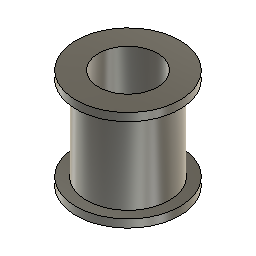
1 x 1 Cable Duct (Autodesk Fusion 360 design; units mm, degrees)
Autodesk Fusion 360 part; units mm, degrees
sketch "Walls" plane through (0, 0, 0) normal (0, 1, 0) x (1, 0, 0)
  line L0 (0, 0) -> (0, -25.4) construction
  line L1 (10.646, 2.4) -> (10.646, -25.4)
  line L2 (10.646, -25.4) -> (12.446, -25.4)
  line L3 (12.446, -25.4) -> (12.446, 0)
  line L4 (12.446, 0) -> (15.621, 0)
  line L5 (15.621, 0) -> (15.621, 2.4)
  line L6 (15.621, 2.4) -> (10.646, 2.4)
  line L7 (10.646, 2.4) -> (8.846, 2.4)
  line L8 (8.846, 2.4) -> (8.846, -27.8)
  line L9 (8.846, -27.8) -> (15.621, -27.8)
  line L10 (15.621, -27.8) -> (15.621, -25.4)
  line L11 (15.621, -25.4) -> (10.646, -25.4)
  line L12 (10.646, 1.2) -> (11.846, 0)
  line L13 (11.846, 0) -> (10.646, -1.2)
  dimension "d56" = 25.4
  dimension "d57" = 2.4
  dimension "d58" = 1.8
  dimension "d59" = 12.446
  dimension "d60" = 3.175
  dimension "d61" = 1.2
  dimension "d62" = 1.2
  constraint parallel L0 L1
  constraint perpendicular L0 L2
  constraint perpendicular L2 L3
  constraint perpendicular L0 L4
  constraint perpendicular L4 L5
  constraint horizontal L6
  constraint coincident L0.start origin
  constraint coincident L0.end L2
  constraint perpendicular L1 L7
  constraint perpendicular L6 L8
  constraint perpendicular L1 L9
  constraint perpendicular L9 L10
  constraint collinear L5 L10
  constraint equal L5 L10
  constraint horizontal L11
  constraint coincident L1 L12.start
  constraint coincident L1 L13.end
  constraint equal L12 L13
  constraint perpendicular L12 L13
  constraint coincident L0.start L4
  measures "d56" distance of L0.start L0.end
  measures "d57" distance of L4.end L5.end
  measures "d58" distance of L1.end L2.end
  measures "d59" distance of L0 L3
  measures "d60" distance of L3.end L4.end
  measures "d61" distance of L1.start L12.start
  measures "d62" distance of L1 L12.end
revolve "Revolve1" add sketch "Walls" angle 360 about axis through (0, 0, 0) along (0, 0, 1) contours L1 L2 L3 L4 L5 L6 L11 L12 L13 makes body 1 in component "Outer"
revolve "Revolve1'" add sketch "Walls" angle 360 about axis through (0, 0, 0) along (0, 0, 1) separate body contours L1 L2 L7 L8 L9 L10 L11 | L1 L12 L13 makes body 2 in component "Inner"
move_face "OffsetFaces1" offset -0.127 5 faces at (10.6328, -0.5307, 9.2667) (11.4318, -0.5705, 0.4) (11.3891, -1.1397, -0.4) (10.5931, -1.06, -1.6) (9.9734, -0.9684, -2.4) on bodies 2 in component "Inner"
sketch "Cutouts" plane through (0, 0, -2.273) normal (0, 0, -1) x (1, 0, 0)
  circle A0 centre (0, 0) radius 8.846
  circle A1 centre (0, 0) radius 10.519
  circle A2 centre (0, 0) radius 8.846 construction
  circle A3 centre (0, 0) radius 15.621 construction
  line L0 (-1.2, 15.621) -> (1.2, 15.621)
  line L1 (1.2, 15.621) -> (1.2, 8.7642)
  line L2 (1.2, 8.7642) -> (-1.2, 8.7642)
  line L3 (-1.2, 8.7642) -> (-1.2, 15.621)
  line L4 (0, 0) -> (0, 8.846) construction
  dimension "d66" = 2.4
  constraint horizontal L0
  constraint vertical L1
  constraint horizontal L2
  constraint vertical L3
  constraint coincident A0.centre A1.centre
  constraint coincident A2 L4.end
  constraint perpendicular L2 L4
  constraint tangent A3 L0
  constraint coincident A2 L2.end
  measures "d66" distance of L0.start L0.end
extrude "Extrude1" cut sketch "Cutouts" against normal blind 12.7 contours A0 L2 | A0 A1 L1 L3 | A1 L0 L1 L3 picked at (0.1337, 8.7885) picked at (-0.9337, 9.3505) bodies 2 in component "Inner"
pattern_circular "C-Pattern1" count 6 over 360 about axis through (0, 0, 0) along (0, 0, 1) of "Extrude1" in component "Inner"
component "Outer" placed x (1, 0, 0) y (0, 1, 0) z (0, 0, 1) at (0, 0, 0)
component "Inner" placed x (1, 0, 0) y (0, 1, 0) z (0, 0, 1) at (0, 0, 0)
equation "DIAMETER = 1 in - 0.02 in" comment "Diameter of ducting"
equation "LENGTH = 1 in" comment "Thickness flange to flange"
equation "PRINTER_TOLERANCE = 0.005 in" comment "Tolerance for printer"
equation "FLANGE = 0.125 in"
equation "SLOT_WIDTH = 2.4 mm" comment "Width of slots for flange flexibility"
equation "SLOT_DEPTH = LENGTH * 0.5" comment "Depth of slot from flange"
equation "FLANGE_THICKNESS = 2.4 mm" comment "Thickness of flange top and bottom"
equation "FLANGE_OVERHANGE = 45 deg" comment "Angle of the compliant flange side"
equation "WALL = 1.8 mm" comment "Interior wall"
equation "SLOT_COUNT = 6" comment "# of flex slots"
equation "d56 = LENGTH"
equation "d57 = FLANGE_THICKNESS"
equation "d58 = WALL"
equation "d59 = DIAMETER / 2"
equation "d60 = FLANGE"
equation "d61 = WALL / 3 * 2"
equation "d62 = WALL * 2 / 3"
equation "d65 = -PRINTER_TOLERANCE"
equation "d66 = SLOT_WIDTH"
equation "d67 = -SLOT_DEPTH"
equation "d69 = SLOT_COUNT"
